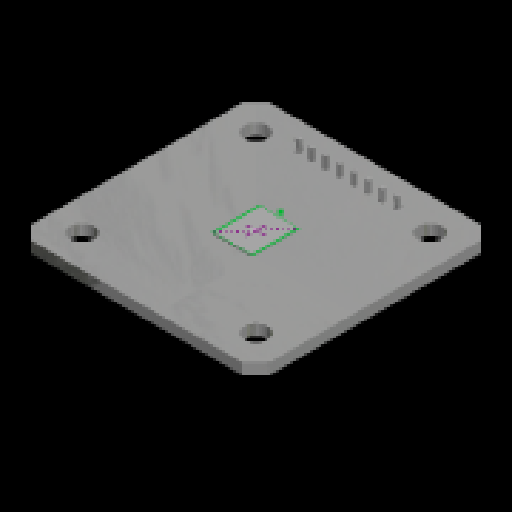
# Autodesk Inventor part: ArmEncoderBoard2
Saved by Autodesk Inventor 2025.2 (Build 292293000, 293)
## iProperties
Created: 2024-03-09
Part Number: ArmEncoderBoard2
Material: Generic
Document SubType Name: Modeling
Designer: valer
Density: 1 g/cm^3
Appearance: Default
Author: valer
Autodesk Inventor part; units mm, degrees
ref_plane "YZ Plane" through (0, 0, 0) normal (1, 0, 0) x (0, 1, 0)
ref_plane "XZ Plane" through (0, 0, 0) normal (0, 1, 0) x (-1, 0, 0)
ref_plane "Work Plane1" through (-14.5282, -0.6229, 20.934) normal (0, 1, 0) x (-1, 0, 0)
sketch "Sketch1" plane through (-14.5282, -0.6229, 20.934) normal (0, 1, 0) x (-1, 0, 0)
  line L0 (-12.2033, -20.3154) -> (-17.7585, -20.3154)
  line L1 (-17.7585, -20.3154) -> (-17.7585, -13.6964)
  line L2 (-17.7585, -13.6964) -> (-12.2033, -13.6964)
  line L3 (-12.2033, -13.6964) -> (-12.2033, -20.3154)
  point P0 (-14.5282, -20.934)
  constraints: 8 end point, 2 parallel, 1 horizontal, 1 perpendicular
extrude "Extrusion1" add sketch "Sketch1" along normal blind 0.25
sketch "Sketch2" plane through (-14.5282, -0.3729, 20.934) normal (0, 1, 0) x (1, 0, 0)
  line L0 (12.2033, 13.6964) -> (17.7585, 13.6964) construction
  line L1 (17.7585, 13.6964) -> (17.7585, 20.3154) construction
  line L2 (17.7585, 20.3154) -> (12.2033, 20.3154) construction
  line L3 (12.2033, 20.3154) -> (12.2033, 13.6964) construction
  line L4 (17.7585, 13.6964) -> (17.7585, 20.3154) projected
  line L5 (12.2033, 20.3154) -> (12.2033, 13.6964) projected
  line L6 (17.7585, 20.3154) -> (12.2033, 13.6964) construction
  point P0 (14.5282, 20.934)
  point P1 (14.9809, 17.0059)
  constraints: 2 end point, 1 midpoint
body "Solid1"
